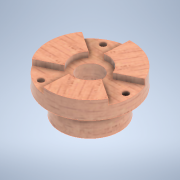
# Autodesk Inventor part: P01_Marcos_Uriel_Martinez_Ortiz2
Saved by Autodesk Inventor 2021 (Build 250183000, 183)
## iProperties
Created: 2021-03-12
Part Number: P01_Marcos_Uriel_Martinez_Ortiz2
Material: Steel ASTM A36
Document SubType Name: Modeling
Designer: uriel
Mass: 607.906 g
Surface Area: 162.239 cm^2
Volume: 77.4402 cm^3
Density: 7.85 g/cm^3
Appearance: White Oak - Natural Medium Gloss
Author: uriel
Autodesk Inventor part; units mm, degrees
ref_plane "YZ Plane" through (0, 0, 0) normal (1, 0, 0) x (0, 1, 0)
ref_plane "XZ Plane" through (0, 0, 0) normal (0, 1, 0) x (-1, 0, 0)
ref_plane "XY Plane" through (0, 0, 0) normal (0, 0, 1) x (1, 0, 0)
sketch "Sketch1" plane through (0, 0, 0) normal (0, 0, 1) x (1, 0, 0)
  line L0 (10, 0) -> (35, 0)
  line L1 (35, 0) -> (35, -10)
  line L2 (35, -10) -> (25, -10)
  line L3 (25, -10) -> (25, -30)
  line L4 (25, -30) -> (10, -30)
  line L5 (10, -30) -> (10, 0)
  line L6 (0, 0) -> (0, -47.182838) construction
  dimension "d0" = 10
  dimension "d1" = 20
  dimension "d2" = 35
  dimension "d3" = 10
  dimension "d4" = 10
  dimension "d5" = 0
  constraints: 14 end point, 3 horizontal, 3 perpendicular, 1 vertical
  measures "d0" distance of L0.end L1.end
  measures "d1" distance of L2.end L3.end
  measures "d2" distance between parallel lines of L1 L6
  measures "d3" distance of L1.end L2.end
  measures "d4" distance between parallel lines of L6 L5
  measures "d5" distance from line of L6.start L0
sketch "Sketch1 outline for Revolution1" plane through (0, 0, 0) normal (0, 0, 1) x (1, 0, 0)
  line L0 (10, 0) -> (10, -30)
  line L1 (35, 0) -> (10, 0)
  line L2 (35, -10) -> (35, 0)
  line L3 (25, -10) -> (35, -10)
  line L4 (25, -30) -> (25, -10)
  line L5 (10, -30) -> (25, -30)
revolve "Revolution1" add sketch "Sketch1 outline for Revolution1" angle 360 about axis through (0, 0, 0) along (0, -1, 0)
sketch "Sketch2" plane through (0, 0, 0) normal (0, 1, 0) x (-1, 0, 0)
  circle A0 centre (0, 0) radius 35
  arc A1 (11.18034, -10) -> (11.18034, 10) centre (0, 0) ccw
  line L0 (11.18034, 10) -> (29.349814, 19.067995)
  circle A2 centre (0, 0) radius 35
  line L1 (11.18034, -10) -> (27.938175, -21.082182)
  arc A3 (27.977577, -21.108239) -> (29.6661, 19.225846) centre (0, 0.265385) ccw
  circle A4 centre (0, 0) radius 10
  dimension "d7" = 30
  dimension "d8" = 60
  constraints: 6 point on circle, 4 end point, 2 centre point, 2 point on line, 1 coincident, 1 concentric
  measures "d7" diameter of A1
  measures "d8" angle of L1 L0
sketch "Sketch2 outline for Extrusion1" plane through (0, 0, 0) normal (0, 1, 0) x (-1, 0, 0)
  arc A0 (11.18034, 10) -> (11.18034, -10) centre (0, 0) cw
  line L0 (29.349814, 19.067995) -> (11.18034, 10)
  arc A1 (27.938175, -21.082182) -> (29.349814, 19.067995) centre (0, 0) ccw
  line L1 (11.18034, -10) -> (27.938175, -21.082182)
extrude "Extrusion1" add sketch "Sketch2 outline for Extrusion1" along normal blind 5
sketch "Sketch3" plane through (0, 0, 0) normal (0, 1, 0) x (-1, 0, 0)
  circle A0 centre (-30, 0) radius 2.5
  point P0 (0, 0)
  dimension "d11" = 5
  dimension "d12" = 30
  constraints: 1 centre point
  measures "d11" diameter of A0
  measures "d12" distance of A0.centre point (0, 0)
sketch "Sketch3 outline for Extrusion2" plane through (0, 0, 0) normal (0, 1, 0) x (-1, 0, 0)
  circle A0 centre (-30, 0) radius 2.5
extrude "Extrusion2" cut sketch "Sketch3 outline for Extrusion2" against normal blind 10
pattern_circular "Circular Pattern1" count 3 over 360 about axis through (0, -15, 0) along (0, -1, 0) of "Extrusion1"
pattern_circular "Circular Pattern2" count 3 over 360 about axis through (0, -15, 0) along (0, -1, 0) of "Extrusion2"
body "Solid1"
